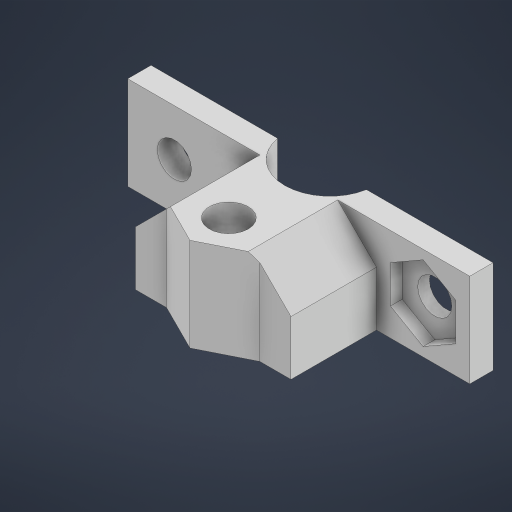
# Autodesk Inventor part: mounter_top
Saved by Autodesk Inventor 2023 (Build 270158000, 158)
## iProperties
Created: 2023-03-04
Part Number: mounter_top
Material: 一般
Document SubType Name: Modeling
Designer: neko2
Density: 1 g/cm^3
Appearance: 既定
Author: neko2
Autodesk Inventor part; units mm, degrees
ref_plane "YZ Plane" through (0, 0, 0) normal (1, 0, 0) x (0, 1, 0)
ref_plane "XZ Plane" through (0, 0, 0) normal (0, 1, 0) x (-1, 0, 0)
ref_plane "XY Plane" through (0, 0, 0) normal (0, 0, 1) x (1, 0, 0)
sketch "スケッチ1" plane through (0, 0, 0) normal (0, 1, 0) x (-1, 0, 0)
  line L0 (15, 2.5) -> (-15, 2.5)
  line L1 (-15, 2.5) -> (-15, -2.5)
  line L2 (-15, -2.5) -> (15, -2.5)
  line L3 (15, -2.5) -> (15, 2.5)
  line L4 (15, 2.5) -> (-15, -2.5) construction
  line L5 (-15, 2.5) -> (15, -2.5) construction
  point P0 (0, 0)
  dimension "d0" = 30
  dimension "d1" = 5
  constraints: 12 end point, 2 midpoint, 2 parallel, 1 horizontal, 1 perpendicular
  measures "d0" distance of L2.end L1.end
  measures "d1" distance of L1.end L0.end
extrude "押し出し1" add sketch "スケッチ1" along normal blind 7
sketch "スケッチ2" plane through (0, 7, 0) normal (0, 1, 0) x (1, 0, 0)
  circle A0 centre (0, 12.5) radius 2.9
  circle A1 centre (0, 12.5) radius 5.3852
  line L0 (-11, 10.5) -> (-5, 10.5)
  line L1 (-5, 10.5) -> (-5, 2.5)
  line L2 (15, 2.5) -> (-15, 2.5) projected
  line L3 (0, -8.1348) -> (0, 42.7212)
  line L4 (-15, -2.5) -> (15, -2.5) projected
  line L5 (15, -2.5) -> (15, 2.5) projected
  line L6 (15, 2.5) -> (-15, 2.5) projected
  line L7 (-15, 2.5) -> (-15, -2.5) projected
  line L8 (-15, -2.5) -> (15, -2.5) projected
  line L9 (-11, 10.5) -> (-11, 12)
  line L10 (-11, 12) -> (0, 12)
  line L11 (11, 10.5) -> (5, 10.5)
  line L12 (5, 10.5) -> (5, 2.5)
  line L13 (11, 10.5) -> (11, 12)
  line L14 (11, 12) -> (0, 12)
  point P0 (0, 0)
  point P1 (2.8566, 12)
  point P2 (-2.8566, 12)
  dimension "d5" = 5.8
  dimension "d9" = 6
  dimension "d10" = 10
  dimension "d40" = 0.5
  dimension "d41" = 15
  dimension "d42" = 1.5
  constraints: 18 end point, 4 point on line, 4 symmetric about line, 3 vertical, 2 perpendicular, 1 centre point, 1 coincident, 1 vertical alignment, 3 other
  measures "d5" diameter of A0
  measures "d9" distance of L0.start L0.end
  measures "d10" distance of L2.end L1.end
  measures "d40" distance of L10.end A0.centre
  measures "d41" horizontal distance of L4.start A0.centre
  measures "d42" distance of L0.start L9.end
extrude "押し出し2" add sketch "スケッチ2" along normal blind 6 contours L14 A1 L3 A0 | A0 L3 A1 L10 | L14 L13 L11 A1 | A1 L0 L9 L10 | L3 L2 L1 A1 | A1 L12 L2 L3 | L3 L4 L7 L2 | L2 L5 L4 L3 picked at (0.6464, 8.0199) picked at (-0.6464, 8.0199)
sketch "スケッチ4" plane through (0, 0, 0) normal (0, -1, 0) x (1, 0, 0)
  line L0 (-15, 2.5) -> (15, 2.5) projected
  line L1 (-15, -2.5) -> (-15, 2.5) projected
  line L2 (-15, 2.5) -> (15, 2.5) projected
  circle A0 centre (-12.5, 0) radius 1.6
  line L3 (0, 2.5) -> (0, -2.5)
  circle A1 centre (12.5, 0) radius 1.6
  point P0 (0, 0)
  point P1 (-15, 0)
  dimension "d78" = 3.2
  dimension "d79" = 2.5
  constraints: 2 centre point, 2 end point, 2 midpoint, 1 horizontal alignment, 1 symmetric about line, 1 vertical, 1 other
  measures "d78" diameter of A0
  measures "d79" distance from line of L1 A0.centre
extrude "押し出し4" cut sketch "スケッチ4" against normal blind 5
sketch "スケッチ5" plane through (-11, 7, -10.5) normal (0, 0, 1) x (1, 0, 0)
  circle A0 centre (3, 3) radius 1.1
  circle A1 centre (19, 3) radius 1.1
  line L0 (0, 6) -> (6, 6) projected
  line L1 (0, 0) -> (0, 6) projected
  line L2 (19, 5.3) -> (17, 4.1528)
  line L3 (17, 4.1528) -> (17, 1.8472)
  line L4 (17, 1.8472) -> (19, 0.7)
  line L5 (19, 0.7) -> (21, 1.8472)
  line L6 (21, 1.8472) -> (21, 4.1528)
  line L7 (21, 4.1528) -> (19, 5.3)
  line L8 (17, 1.8472) -> (21, 4.1528)
  line L9 (17, 4.1528) -> (21, 1.8472)
  line L10 (19, 5.3) -> (19, 0.7)
  line L11 (16.9, 4.2107) -> (19, 5.4153)
  line L12 (19, 5.4153) -> (21.1, 4.2107)
  line L13 (21.1, 4.2107) -> (21.1, 1.7893)
  line L14 (21.1, 1.7893) -> (19, 0.5847)
  line L15 (19, 0.5847) -> (16.9, 1.7893)
  line L16 (16.9, 1.7893) -> (16.9, 4.2107)
  line L17 (16, 6) -> (22, 6) projected
  line L18 (22, 0) -> (22, 6) projected
  point P0 (11, -7)
  point P1 (3, 6)
  point P2 (0, 3)
  point P3 (19, 6)
  point P4 (22, 3)
  dimension "d0" = 30
  dimension "d1" = 5
  dimension "d27" = 2.2
  dimension "d28" = 2.2
  dimension "d29" = 4.6
  dimension "d31" = 4
  dimension "d35" = 0.1
  constraints: 30 end point, 8 midpoint, 5 equal length, 3 parallel, 3 vertical alignment, 2 centre point, 2 horizontal alignment, 1 point on line, 1 vertical, 5 other
  measures "d27" diameter of A0
  measures "d28" diameter of A1
  measures "d29" distance of L4.end L2.start
  measures "d31" distance between parallel lines of L6 L3
  measures "d35" distance between parallel lines of L2 L11
extrude "押し出し5" cut sketch "スケッチ5" against normal blind 0.75 contours A1 L9 L8 | A1 L8 L6 L9 | L8 L10 A1 | A1 L10 L7 L8 | L9 L5 L10 A1 | A1 L10 L9 | L10 L9 A1 | A1 L9 L2 L10 | L10 A1 L8 | L8 A1 L9 | L10 L4 L8 A1 | A1 L8 L3 L9 | L11 L12 L13 L14 L15 L16
extrude "押し出し6" cut sketch "スケッチ5" against normal through all contours A0
extrude "押し出し7" cut sketch "スケッチ5" against normal through all contours A1 L9 L8 | L8 L10 A1 | A1 L10 L9 | L10 L9 A1 | L10 A1 L8 | L8 A1 L9
sketch "スケッチ7" plane through (15, 0, -2.5) normal (0, 0, -1) x (-1, 0, 0)
  line L0 (10, 7.5) -> (0, 7.5)
  line L1 (0, 0) -> (0, 13) projected
  line L2 (10, 13) -> (10, 7.5)
  circle A0 centre (7, 10) radius 1.1 projected
  line L3 (4, 7) -> (12.1434, 7) projected
  line L4 (12.1434, 7) -> (12.1434, 13) projected
  line L5 (4, 13) -> (12.1434, 13) projected
  line L6 (4, 7) -> (4, 13) projected
  line L7 (0, 0) -> (30, 0) projected
  line L8 (30, 0) -> (30, 13) projected
  line L9 (20, 13) -> (30, 13) projected
  line L10 (20, 7) -> (20, 13) projected
  line L11 (10, 7) -> (20, 7) projected
  line L12 (10, 7) -> (10, 13) projected
  line L13 (0, 13) -> (10, 13) projected
  line L14 (0, 0) -> (0, 13) projected
  line L15 (15, 13) -> (15, 0)
  line L16 (20, 7.5) -> (30, 7.5)
  line L17 (20, 13) -> (20, 7.5)
  dimension "d53" = 0.5
  constraints: 10 end point, 3 symmetric about line, 2 perpendicular, 1 point on line, 1 vertical
  measures "d53" distance between parallel lines of L0 L3
extrude "押し出し8" cut sketch "スケッチ7" against normal through all contours L0 L6 L5 L2 | L0 L1 L13 L6 | L10 L9 L8 L16 | A0
chamfer "面取り6" distance 3 angle 45 2 edges at (5, 7.5, 0) (-5, 7.5, 0)
chamfer "面取り7" distance 2 angle 45 2 edges at (15, 7.5, 0) (-15, 7.5, 0)
chamfer "面取り8" distance 2.5 angle 45 2 edges at (5, 13, -4) (-5, 13, -4)
chamfer "面取り9" distance 2 angle 45 11 edges at (-10.5, 7.5, 2.5) (-6.5, 9, 2.5) (0, 13, 2.5) (6.5, 9, 2.5) (10.5, 7.5, 2.5) (-14, 6.5, -2.5) (-10.5, 7.5, -2.5) (-6.5, 9, -2.5) (6.5, 9, -2.5) (10.5, 7.5, -2.5) (14, 6.5, -2.5)
sketch "スケッチ9" plane through (0, 13, 0) normal (0, 1, 0) x (1, 0, 0)
  circle A0 centre (0, 6) radius 1.25
  point P0 (0, 0)
  dimension "d74" = 2.5
  dimension "d75" = 6
  constraints: 1 centre point, 1 vertical alignment
  measures "d74" diameter of A0
  measures "d75" distance of point (0, 0) A0.centre
extrude "押し出し9" cut sketch "スケッチ9" against normal through all
sketch "スケッチ10" plane through (0, 7, 0) normal (0, -1, 0) x (1, 0, 0)
  line L0 (5, -2.5) -> (5, -10.5) projected
  line L1 (5, -5) -> (3, -5)
  line L2 (3, -5) -> (0, -3.5)
  line L3 (0, -3.5) -> (-3, -5)
  line L4 (-3, -5) -> (-5, -5)
  line L5 (15, -2.5) -> (-15, -2.5) projected
  line L6 (-5, -10.5) -> (-5, -2.5) projected
  point P0 (0, 0)
  dimension "d80" = 2.5
  dimension "d81" = 1.5
  dimension "d82" = 2
  constraints: 8 end point, 2 equal length, 2 horizontal, 2 point on line, 1 horizontal alignment
  measures "d80" distance from line of L1.start L5
  measures "d81" vertical distance of L2.end L1.end
  measures "d82" distance of L1.start L1.end
split body "分割2" sketch "スケッチ10" result one side removed curves L1 L2 L3 L4 removed pieces at (2.3905, 1.8333, 2)
